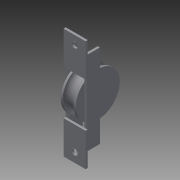
# Autodesk Inventor part: 知能ロボコンショウレックス戸草
Saved by Autodesk Inventor 2013 (Build 170138000, 138)
## iProperties
Created: 2014-05-28
Part Number: 知能ロボコンショウレックス戸草
Material: 一般
Document SubType Name: Modeling
Designer: horumo136
Density: 1 g/cm^3
Author: horumo136
Autodesk Inventor part; units mm, degrees
ref_plane "YZ Plane" through (0, 0, 0) normal (1, 0, 0) x (0, 1, 0)
ref_plane "XZ Plane" through (0, 0, 0) normal (0, 1, 0) x (-1, 0, 0)
ref_plane "XY Plane" through (0, 0, 0) normal (0, 0, 1) x (1, 0, 0)
sketch "スケッチ1" plane through (0, 0, 0) normal (0, 0, 1) x (1, 0, 0)
  line L0 (0, 0) -> (8.2, 0)
  line L1 (8.2, 0) -> (4.1, 0)
  line L2 (0, 0) -> (0, 12)
  line L3 (8.2, 0) -> (8.2, 12)
  line L4 (4.1, 0) -> (4.1, 9.65)
  line L5 (0, 12) -> (1.1, 12)
  line L6 (8.2, 12) -> (7.1, 12)
  arc A0 (1.1, 12) -> (7.1, 12) centre (4.1, 12.7399) ccw
  dimension "d0" = 8.2
  dimension "d1" = 12
  dimension "d2" = 12
  dimension "d3" = 9.65
  dimension "d4" = 1.1
  dimension "d5" = 1.1
  constraints: 14 end point, 3 point on circle, 2 parallel, 2 perpendicular, 1 centre point, 1 collinear, 1 horizontal, 1 midpoint
  measures "d0" distance of L0.start L0.end
  measures "d1" distance of L0.start L2.end
  measures "d2" distance of L0.end L3.end
  measures "d3" distance of L1.end L4.end
  measures "d4" distance of L2.end L5.end
  measures "d5" distance of L3.end L6.end
revolve "回転1" add sketch "スケッチ1" angle 360 about axis through (0, 0, 0) along (1, 0, 0)
sketch "スケッチ2" plane through (8.2, 0, 0) normal (1, 0, 0) x (0, 0, -1)
  circle A0 centre (0, 0) radius 12 projected
  line L0 (0, 0) -> (22.8, 0)
  line L1 (0, 0) -> (0, -7.2)
  line L2 (0, 0) -> (22.8, 0)
  line L3 (22.8, 0) -> (22.8, -7.2)
  line L4 (22.8, -7.2) -> (0, -7.2)
  line L5 (0, -7.2) -> (0, 0)
  line L6 (0, 0) -> (-22.8, 0)
  line L7 (-22.8, 0) -> (-22.8, -7.2)
  line L8 (-22.8, -7.2) -> (0, -7.2)
  dimension "d7" = 22.8
  dimension "d8" = 7.2
  dimension "d17" = 0
  constraints: 18 end point, 2 horizontal, 2 parallel, 2 perpendicular, 2 symmetric about line
  measures "d7" distance of L0.start L0.end
  measures "d8" distance of L0.start L1.end
  measures "d17" distance from line of L3 L0.end
extrude "押し出し1" add sketch "スケッチ2" along normal blind 1.2 contours L0 L3 L4 A0 | A0 L4 L1 L0 | L6 L1 L8 A0 | A0 L8 L7 L6
sketch "スケッチ3" plane through (0, 0, 0) normal (-1, 0, 0) x (0, 0, 1)
  circle A0 centre (0, 0) radius 12 projected
  line L0 (0, 0) -> (0, -7.2)
  line L1 (0, -7.2) -> (22.8, -7.2)
  line L2 (0, 0) -> (22.8, 0)
  line L3 (22.8, 0) -> (22.8, -7.2)
  line L4 (22.8, -7.2) -> (0, -7.2)
  line L5 (0, -7.2) -> (0, 0)
  line L6 (0, 0) -> (-22.8, 0)
  line L7 (-22.8, 0) -> (-22.8, -7.2)
  line L8 (-22.8, -7.2) -> (0, -7.2)
  dimension "d11" = 7.2
  dimension "d12" = 22.8
  constraints: 18 end point, 2 parallel, 2 perpendicular, 2 symmetric about line, 1 horizontal, 1 vertical
  measures "d11" distance of L0.start L0.end
  measures "d12" distance of L0.end L1.end
extrude "押し出し2" add sketch "スケッチ3" along normal blind 2 contours L2 L3 L1 A0 | A0 L1 L0 L2 | L6 L0 L8 A0 | A0 L8 L7 L6
sketch "スケッチ4" plane through (-2, 0, 0) normal (-1, 0, 0) x (0, 0, 1)
  line L0 (-22.8, -7.2) -> (22.8, -7.2) projected
  line L1 (0, -7.2) -> (12.1, -7.2)
  line L2 (12.1, -7.2) -> (30.2, -7.2)
  line L3 (12.1, -7.2) -> (30.2, -7.2)
  line L4 (30.2, -7.2) -> (30.2, -8.4)
  line L5 (30.2, -8.4) -> (12.1, -8.4)
  line L6 (12.1, -8.4) -> (12.1, -7.2)
  line L7 (0, 0) -> (0, -1.8874)
  line L8 (-12.1, -7.2) -> (-30.2, -7.2)
  line L9 (-30.2, -7.2) -> (-30.2, -8.4)
  line L10 (-30.2, -8.4) -> (-12.1, -8.4)
  line L11 (-12.1, -8.4) -> (-12.1, -7.2)
  dimension "d15" = 12.1
  dimension "d16" = 18.1
  dimension "d18" = 1.2
  constraints: 22 end point, 4 symmetric about line, 3 parallel, 2 point on line, 1 horizontal, 1 midpoint, 1 perpendicular
  measures "d15" distance of L1.start L1.end
  measures "d16" distance of L1.end L2.end
  measures "d18" distance of L3.end L4.end
extrude "押し出し3" add sketch "スケッチ4" against normal blind 12
sketch "スケッチ5" plane through (-2, -8.4, 12.1) normal (0, -1, 0) x (1, 0, 0)
  line L0 (0, 18.1) -> (12, 18.1) projected
  line L1 (6, 18.1) -> (6, 13.4)
  line L2 (6, 13.4) -> (6, -37.2)
  circle A0 centre (6, -37.2) radius 1.6
  circle A1 centre (6, 13.4) radius 1.6
  point P0 (2, -12.1)
  dimension "d21" = 4.7
  dimension "d22" = 50.6
  dimension "d23" = 3.2
  dimension "d24" = 3.2
  constraints: 4 end point, 2 centre point, 2 coincident, 1 collinear, 1 midpoint, 1 perpendicular
  measures "d21" distance of L1.start L1.end
  measures "d22" distance of L1.end L2.end
  measures "d23" diameter of A0
  measures "d24" diameter of A1
hole "穴1" at (4, -8.4, 25.5) at (4, -8.4, -25.1) direction (0, 1, 0) diameter 3.2 depth 8 tip angle 118
